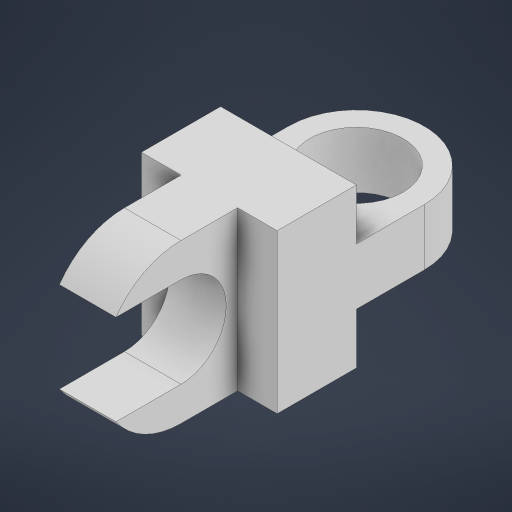
# Autodesk Inventor part: Część19
Saved by Autodesk Inventor 2023 (Build 270158000, 158)
## iProperties
Created: 2023-05-08
Part Number: Część19
Material: Ogólny
Document SubType Name: Modeling
Designer: Adam
Density: 1 g/cm^3
Appearance: Domyślna
Author: Adam
Autodesk Inventor part; units mm, degrees
ref_plane "YZ Plane" through (0, 0, 0) normal (1, 0, 0) x (0, 1, 0)
ref_plane "XZ Plane" through (0, 0, 0) normal (0, 1, 0) x (-1, 0, 0)
ref_plane "XY Plane" through (0, 0, 0) normal (0, 0, 1) x (1, 0, 0)
sketch "Szkic1" plane through (0, 0, 0) normal (0, 1, 0) x (-1, 0, 0)
  line L0 (0, 0) -> (24, 0)
  line L1 (24, 0) -> (24, -14)
  line L2 (24, -14) -> (0, -14)
  line L3 (0, -14) -> (0, 0)
  line L4 (17, 0) -> (7, 0)
  line L5 (7, 0) -> (7, 24)
  line L6 (7, 24) -> (17, 24)
  line L7 (17, 24) -> (17, 0)
  point P0 (7, 0)
  dimension "d0" = 24
  dimension "d1" = 14
  dimension "d2" = 10
  dimension "d3" = 24
  dimension "d4" = 7
  constraints: 16 end point, 4 parallel, 2 horizontal, 2 perpendicular, 1 point on line
  measures "d0" distance of L1.end L2.end
  measures "d1" distance of L0.end L1.end
  measures "d2" distance of L5.end L6.end
  measures "d3" distance of L4.end L5.end
  measures "d4" distance between parallel lines of L3 L5
extrude "Wyciągnięcie proste1" add sketch "Szkic1" along normal blind 28
fillet "Zaokrąglenie1" radius 14 2 edges at (-12, 28, 24) (-12, 0, 24)
sketch "Szkic2" plane through (-7, 0, 0) normal (1, 0, 0) x (0, 0, -1)
  circle A0 centre (-10, 14) radius 8
  line L0 (-10, 0) -> (0, 0) projected
  line L1 (-10, 22) -> (-24, 22)
  line L2 (-24, 22) -> (-24, 6)
  line L3 (-24, 6) -> (-10, 6)
  line L4 (-10, 6) -> (-10, 22)
  dimension "d8" = 16
  dimension "d9" = 14
  constraints: 8 end point, 2 parallel, 1 horizontal, 1 perpendicular, 3 other
  measures "d9" distance from line of L0 point (-10, 14)
extrude "Wyciągnięcie proste2" cut sketch "Szkic2" against normal through all
sketch "Szkic3" plane through (0, 0, -14) normal (0, 0, -1) x (-1, 0, 0)
  line L0 (0, 0) -> (0, 28) projected
  line L1 (24, 0) -> (24, 28) projected
  line L2 (0, 19) -> (24, 19)
  line L3 (24, 19) -> (24, 9)
  line L4 (24, 9) -> (0, 9)
  line L5 (0, 9) -> (0, 19)
  line L6 (0, 28) -> (24, 28) projected
  line L7 (0, 0) -> (24, 0) projected
  point P0 (0, 9)
  dimension "d12" = 9
  dimension "d13" = 9
  constraints: 8 end point, 2 parallel, 2 point on line, 1 horizontal, 1 perpendicular
  measures "d12" distance between parallel lines of L6 L2
  measures "d13" distance between parallel lines of L7 L4
extrude "Wyciągnięcie proste3" add sketch "Szkic3" along normal blind 24 contours L0 L2 L1 L4
full round fillet "Zaokrąglenie pełne1" first side at (0, 12.3333, -4.6667) centre faces at (-8, 15.6667, -38) second side at (-24, 12.3333, -4.6667)
sketch "Szkic4" plane through (-24, 19, -14) normal (0, 1, 0) x (1, 0, 0)
  arc A0 (24, 12) -> (0, 12) centre (12, 12) ccw projected
  point P0 (24, -14)
  constraints: 1 coincident
hole "Otwór1" at (-12, 19, -26) direction (0, -1, 0) diameter 16.5 end through all
